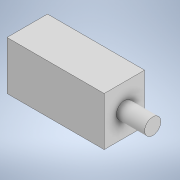
# Autodesk Inventor part: Motor
Saved by Autodesk Inventor 2020 (Build 240168000, 168)
## iProperties
Created: 2021-08-11
Part Number: Motor
Material: Generic
Document SubType Name: Modeling
Designer: Judac
Density: 1 g/cm^3
Appearance: Default
Author: Judac
Autodesk Inventor part; units mm, degrees
ref_plane "YZ Plane" through (0, 0, 0) normal (1, 0, 0) x (0, 1, 0)
ref_plane "XZ Plane" through (0, 0, 0) normal (0, 1, 0) x (-1, 0, 0)
ref_plane "XY Plane" through (0, 0, 0) normal (0, 0, 1) x (1, 0, 0)
sketch "Sketch1" plane through (0, 0, 0) normal (0, 1, 0) x (-1, 0, 0)
  line L0 (0, 0) -> (24, 0)
  line L1 (24, 0) -> (24, -10)
  line L2 (24, -10) -> (0, -10)
  line L3 (0, -10) -> (0, 0)
  dimension "d0" = 24
  dimension "d1" = 10
  constraints: 8 end point, 2 parallel, 1 horizontal, 1 perpendicular
  measures "d0" distance of L0.start L0.end
  measures "d1" distance of L0.end L1.end
extrude "Extrusion1" add sketch "Sketch1" along normal blind 12
sketch "Sketch2" plane through (0, 0, 0) normal (1, 0, 0) x (0, 0, -1)
  circle A0 centre (5, 6) radius 2
  line L0 (10, 0) -> (10, 12) construction
  line L1 (10, 6) -> (0, 6) construction
  line L2 (0, 0) -> (0, 12) construction
  line L3 (10, 12) -> (0, 12) construction
  line L4 (5, 12) -> (5, 0) construction
  line L5 (10, 0) -> (0, 0) construction
  point P0 (5, 6)
  dimension "d4" = 4
  constraints: 5 midpoint, 4 end point, 1 centre point, 1 coincident
  measures "d4" diameter of A0
extrude "Extrusion2" add sketch "Sketch2" along normal blind 7
body "Solid1"
